Slider Rail (Autodesk Fusion 360 design; units mm, degrees)
Autodesk Fusion 360 part; units mm, degrees
sketch "Sketch1" plane through (0, 0, 0) normal (1, 0, 0) x (0, 1, 0)
  line L0 (-10, 0) -> (-10, -35)
  line L1 (-10, -35) -> (100, -35)
  line L2 (100, -35) -> (100, 0)
  line L3 (0, 10) -> (90, 10)
  line L4 (0, 5.5) -> (90, 5.5)
  line L5 (90, -5.5) -> (0, -5.5)
  arc A0 (0, 10) -> (-10, 0) centre (0, 0) ccw
  arc A1 (0, 5.5) -> (0, -5.5) centre (0, 0) ccw
  arc A2 (100, 0) -> (90, 10) centre (90, 0) ccw
  arc A3 (90, -5.5) -> (90, 5.5) centre (90, 0) ccw
  line L6 (-10, -35) -> (-10, -22.5) construction
  line L7 (-10, -22.5) -> (100, -22.5) construction
  line L8 (45, -22.5) -> (45, -35) construction
  circle A4 centre (15, -22.5) radius 2.5
  circle A5 centre (55, -22.5) radius 2.5
  dimension "d1" = 11
  dimension "d2" = 20
  dimension "d3" = 11
  dimension "d4" = 20
  dimension "d5" = 90
  dimension "d7" = 35
  dimension "d10" = 12.5
  dimension "d11" = 5
  dimension "d12" = 5
  dimension "d16" = 30
  dimension "d17" = 10
  constraint coincident A0.centre A1.centre
  constraint concentric A0 A1
  constraint concentric A2 A3
  constraint horizontal A0.centre A2.centre
  constraint tangent L0 A0
  constraint perpendicular L0 L1
  constraint tangent L2 A2
  constraint vertical L2
  constraint vertical L0
  constraint tangent L3 A2
  constraint tangent L3 A0
  constraint tangent L4 A3
  constraint tangent L5 A1
  constraint tangent L5 A3
  constraint tangent L4 A1
  constraint perpendicular L1 L6
  constraint coincident L2 L7.end
  constraint perpendicular L2 L7
  constraint midpoint L7 L8.start
  constraint midpoint L1 L8.end
  constraint coincident L7 A4.centre
  constraint coincident L7 A5.centre
  measures "d1" diameter of A1
  measures "d2" diameter of A0
  measures "d3" diameter of A3
  measures "d4" diameter of A2
  measures "d5" distance of A0.centre A2.centre
  measures "d7" distance of L0.start L0.end
  measures "d10" distance of L0.end L6.end
  measures "d11" diameter of A4
  measures "d12" diameter of A5
  measures "d16" distance of L8.start A4.centre L1.end
  measures "d17" distance of L8.start A5.centre
extrude "Extrude1" add sketch "Sketch1" along normal blind 3.175
fillet "Fillet1" radius 10 1 edges at (1.5875, -10, -35)
fillet "Fillet2" radius 30 1 edges at (1.5875, 100, -35)
